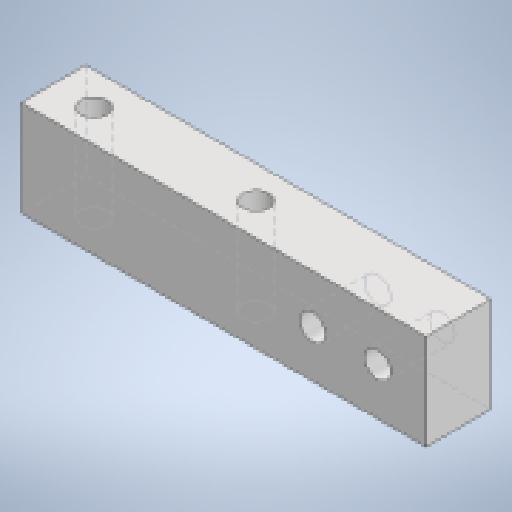
# Autodesk Inventor part: AngleScrewBlocActuator
Saved by Autodesk Inventor 2023 (Build 270158000, 158)
## iProperties
Created: 2023-05-01
Part Number: AngleScrewBlocActuator
Material: Generic
Document SubType Name: Modeling
Designer: Nathann
Density: 1 g/cm^3
Appearance: Default
Author: Nathann
Autodesk Inventor part; units mm, degrees
ref_plane "YZ Plane" through (0, 0, 0) normal (1, 0, 0) x (0, 1, 0)
ref_plane "XZ Plane" through (0, 0, 0) normal (0, 1, 0) x (-1, 0, 0)
ref_plane "XY Plane" through (0, 0, 0) normal (0, 0, 1) x (1, 0, 0)
sketch "Sketch1" plane through (0, 0, 0) normal (0, 0, 1) x (1, 0, 0)
  line L0 (0, 0) -> (-15, 0)
  line L1 (-15, 0) -> (-15, 5.9)
  line L2 (-15, 5.9) -> (0, 5.9)
  line L3 (0, 5.9) -> (0, 0)
  dimension "d0" = 5.9
  dimension "d1" = 15
  constraints: 8 end point, 2 parallel, 1 horizontal, 1 perpendicular
  measures "d0" distance of L0.end L1.end
  measures "d1" distance of L1.end L2.end
extrude "Extrusion1" add sketch "Sketch1" along normal blind 4
sketch "Sketch2" plane through (-15, 5.9, 0) normal (0, 1, 0) x (1, 0, 0)
  circle A0 centre (12.5, -2) radius 0.8
  circle A1 centre (2.5, -2) radius 0.8
  line L0 (15, 0) -> (15, -4) projected
  line L1 (15, -4) -> (0, -4) projected
  dimension "d4" = 10
  dimension "d5" = 2.5
  dimension "d6" = 2
  dimension "d7" = 2
  dimension "d8" = 1.6
  dimension "d9" = 1.6
  constraints: 2 centre point
  measures "d4" distance of A1.centre A0.centre
  measures "d5" distance from line of L0 A0.centre
  measures "d6" distance from line of L1 A0.centre
  measures "d7" distance from line of L1 A1.centre
  measures "d8" diameter of A0
  measures "d9" diameter of A1
extrude "Extrusion2" cut sketch "Sketch2" against normal blind 8
sketch "Sketch3" plane through (0, 0, 0) normal (0, 0, -1) x (-1, 0, 0)
  line L0 (0, 0) -> (0, 5.9) projected
  line L1 (0, 0) -> (-10, 0)
  line L2 (-10, 0) -> (-10, 5.9)
  line L3 (-10, 5.9) -> (0, 5.9)
  line L4 (0, 5.9) -> (0, 0)
  dimension "d12" = 10
  constraints: 8 end point, 2 parallel, 1 horizontal, 1 perpendicular
  measures "d12" distance between parallel lines of L2 L0
extrude "Extrusion3" add sketch "Sketch3" against normal blind 4
sketch "Sketch4" plane through (0, 0, 0) normal (0, 0, -1) x (-1, 0, 0)
  line L0 (3.3, 5.9) -> (3.3, 0) projected
  line L1 (1.7, 5.9) -> (1.7, 0) projected
  circle A0 centre (-3, 1.9) radius 0.8
  circle A1 centre (-7, 1.9) radius 0.8
  line L2 (-10, 5.9) -> (15, 5.9) projected
  line L3 (15, 0) -> (-10, 0) projected
  line L4 (-10, 5.9) -> (-10, 0) projected
  point P0 (0, 0)
  dimension "d15" = 1.6
  dimension "d16" = 5.9
  dimension "d17" = 4
  dimension "d18" = 4
  dimension "d19" = 4
  dimension "d20" = 3
  dimension "d21" = 1.6
  dimension "d22" = 1.6
  constraints: 2 centre point
  measures "d15" distance between parallel lines of L1 L0
  measures "d16" distance between parallel lines of L2 L3
  measures "d17" distance from line of L2 A0.centre
  measures "d18" distance from line of L2 A1.centre
  measures "d19" distance of A1.centre A0.centre
  measures "d20" distance from line of L4 A1.centre
  measures "d21" diameter of A0
  measures "d22" diameter of A1
extrude "Extrusion4" cut sketch "Sketch4" against normal blind 4 contours A0 | A1
equation "\"d7\" = d6"
equation "\"d18\" = d17"
equation "\"d21\" = d15"
equation "\"d22\" = d15"
body "Solid1"
